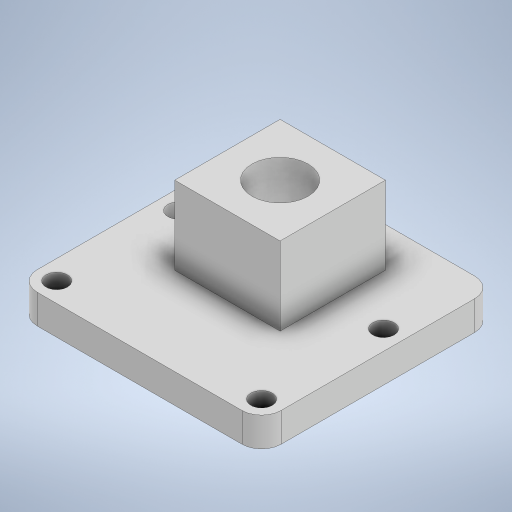
# Autodesk Inventor part: kamera
Saved by Autodesk Inventor 2024.1 (Build 281209000, 209)
## iProperties
Created: 2025-01-07
Part Number: kamera
Material: Všeobecné
Document SubType Name: Modeling
Designer: elias
Density: 1 g/cm^3
Appearance: Výchozí
Author: elias
Autodesk Inventor part; units mm, degrees
ref_plane "YZ Plane" through (0, 0, 0) normal (1, 0, 0) x (0, 1, 0)
ref_plane "XZ Plane" through (0, 0, 0) normal (0, 1, 0) x (-1, 0, 0)
ref_plane "XY Plane" through (0, 0, 0) normal (0, 0, 1) x (1, 0, 0)
sketch "Náčrt1" plane through (0, 0, 0) normal (0, 0, 1) x (1, 0, 0)
  line L0 (12.5, 2) -> (12.5, 21.862)
  line L1 (10.5, 23.862) -> (0, 23.862)
  circle A0 centre (10.5, 2) radius 1.1
  arc A1 (12.5, 3.2809) -> (9.2191, 0) centre (10.5, 2) ccw
  circle A2 centre (10.5, 14.5) radius 1.1
  arc A3 (12.5, 15.7809) -> (12.5, 13.2191) centre (10.5, 14.5) ccw
  line L2 (0, 0) -> (10.5, 0)
  arc A4 (10.5, 0) -> (12.5, 2) centre (10.5, 2) ccw
  arc A5 (12.5, 21.862) -> (10.5, 23.862) centre (10.5, 21.862) ccw
  line L3 (-12.5, 2) -> (-12.5, 21.862)
  line L4 (-10.5, 23.862) -> (0, 23.862)
  circle A6 centre (-10.5, 2) radius 1.1
  arc A7 (-9.2191, 0) -> (-12.5, 3.2809) centre (-10.5, 2) ccw
  circle A8 centre (-10.5, 14.5) radius 1.1
  arc A9 (-12.5, 13.2191) -> (-12.5, 15.7809) centre (-10.5, 14.5) ccw
  line L5 (0, 0) -> (-10.5, 0)
  arc A10 (-12.5, 2) -> (-10.5, 0) centre (-10.5, 2) ccw
  arc A11 (-10.5, 23.862) -> (-12.5, 21.862) centre (-10.5, 21.862) ccw
  dimension "d2" = 2.2
  dimension "d3" = 2
  dimension "d6" = 2.2
  dimension "d8" = 4.75
  dimension "d9" = 2
  dimension "d10" = 23.862
  dimension "d11" = 2
  constraints: 16 point on circle, 12 centre point, 12 end point, 6 point on line, 4 coincident, 3 tangent, 1 horizontal, 1 perpendicular, 1 vertical
  measures "d2" diameter of A0
  measures "d3" distance from line of L0 A0.centre
  measures "d6" diameter of A2
  measures "d8" diameter of A3
  measures "d9" radius of A4
  measures "d10" distance of L2.start L1.end
  measures "d11" radius of A5
extrude "Vysunutí1" add sketch "Náčrt1" along normal blind 3
sketch "Náčrt2" plane through (0, 0, 3) normal (0, 0, 1) x (1, 0, 0)
  line L0 (0, 0) -> (0, 23.862)
  line L1 (10.5, 23.862) -> (-10.5, 23.862) projected
  arc A0 (0, 11.525) -> (0, 17.275) centre (0, 14.4) ccw
  line L2 (-10.5, 0) -> (10.5, 0) projected
  line L3 (-5.4, 9) -> (5.4, 9)
  line L4 (5.4, 9) -> (5.4, 19.8)
  line L5 (5.4, 19.8) -> (-5.4, 19.8)
  line L6 (-5.4, 19.8) -> (-5.4, 9)
  line L7 (-5.4, 9) -> (5.4, 19.8) construction
  line L8 (5.4, 9) -> (-5.4, 19.8) construction
  arc A1 (0, 17.275) -> (0, 11.525) centre (0, 14.4) ccw
  dimension "d14" = 2.875
  dimension "d15" = 14.4
  dimension "d16" = 10.8
  dimension "d17" = 10.8
  constraints: 14 end point, 4 point on circle, 3 midpoint, 3 point on line, 2 centre point, 2 parallel, 1 horizontal, 1 perpendicular, 1 other
  measures "d14" radius of A0
  measures "d15" distance from line of L2 A0.centre
  measures "d16" distance of L3.end L4.end
  measures "d17" distance of L3.start L3.end
extrude "Vysunutí2" add sketch "Náčrt2" along normal blind 8 contours A0 L0 L5 L4 L3 | L0 L3 L6 L5 A1
